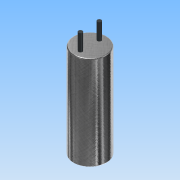
# Autodesk Inventor part: термодатчик
Saved by Autodesk Inventor 2017 (Build 210142000, 142)
## iProperties
Part Number: термодатчик
Material: Типовые
Document SubType Name: Modeling
Designer: Max
Mass: 0.482699 g
Surface Area: 3.87041 cm^2
Volume: 0.482699 cm^3
Density: 1 g/cm^3
Appearance: Лощеная
Author: Max
Autodesk Inventor part; units mm, degrees
ref_plane "YZ Plane" through (0, 0, 0) normal (1, 0, 0) x (0, 1, 0)
ref_plane "XZ Plane" through (0, 0, 0) normal (0, 1, 0) x (-1, 0, 0)
ref_plane "XY Plane" through (0, 0, 0) normal (0, 0, 1) x (1, 0, 0)
sketch "Эскиз1" plane through (0, 0, 0) normal (0, 0, 1) x (1, 0, 0)
  circle A0 centre (0, 0) radius 3
  circle A1 centre (0, 1.6837) radius 0.3522
  circle A2 centre (0, -1.7307) radius 0.3546
  dimension "d0" = 6
  constraints: 3 centre point, 1 coincident
  measures "d0" diameter of A0
extrude "Выдавливание1" add sketch "Эскиз1" against normal blind 17 contours A0 | A1 | A2
extrude "Выдавливание2" add sketch "Эскиз1" along normal blind 3 contours A1 | A2
fillet "Сопряжение1" radius 0.2 2 edges at (-3, 0, 0) (-3, 0, -17)
